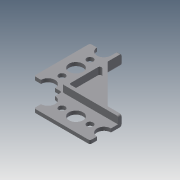
# Autodesk Inventor part: Деталь
Saved by Autodesk Inventor 2014 (Build 180170000, 170)
## iProperties
Created: 2015-11-19
Part Number: Деталь
Material: Типовые
Document SubType Name: Modeling
Designer: 151-362
Density: 1 g/cm^3
Appearance: По умолчанию
Author: 151-362
Autodesk Inventor part; units mm, degrees
ref_plane "YZ Plane" through (0, 0, 0) normal (1, 0, 0) x (0, 1, 0)
ref_plane "XZ Plane" through (0, 0, 0) normal (0, 1, 0) x (-1, 0, 0)
sketch "Эскиз1" plane through (0, 0, 0) normal (0, 0, 1) x (1, 0, 0)
  line L0 (0, 16) -> (0, 48)
  line L1 (0, 48) -> (4, 48)
  arc A0 (4, 48) -> (12, 48) centre (8, 48) ccw
  line L2 (12, 48) -> (18, 48)
  line L3 (18, 48) -> (18, 40)
  line L4 (18, 40) -> (40, 18)
  line L5 (40, 18) -> (48, 18)
  line L6 (48, 18) -> (48, 12)
  arc A1 (48, 12) -> (48, 4) centre (48, 8) ccw
  line L7 (48, 4) -> (48, 0)
  line L8 (48, 0) -> (16, 0)
  line L9 (16, 0) -> (16, 4)
  arc A2 (16, 4) -> (16, 12) centre (16, 8) ccw
  line L10 (16, 12) -> (16, 16)
  line L11 (16, 16) -> (12, 16)
  arc A3 (12, 16) -> (4, 16) centre (8, 16) ccw
  line L12 (0, 16) -> (4, 16)
  circle A4 centre (8, 24) radius 1.85
  circle A5 centre (8, 32) radius 4
  circle A6 centre (8, 40) radius 1.85
  circle A7 centre (40, 8) radius 1.85
  circle A8 centre (32, 8) radius 4
  circle A9 centre (24, 8) radius 1.85
  constraints: 26 end point, 10 centre point, 8 point on circle
extrude "Выдавливание1" add sketch "Эскиз1" along normal blind 2
fillet "Сопряжение1" radius 1 8 edges at (0, 48, 1) (18, 44, 0) (29, 29, 0) (44, 18, 0) (48, 0, 1) (16, 0, 1) (16, 16, 1) (0, 16, 1)
ref_plane "РабПлоскость1" through (0, 0, 2) normal (0, 0, 1) x (1, 0, 0)
sketch "Эскиз2" plane through (0, 0, 2) normal (0, 0, 1) x (1, 0, 0)
  line L0 (16, 16) -> (16, 48)
  line L1 (16, 48) -> (18, 48)
  line L2 (18, 48) -> (18, 40)
  line L3 (18, 40) -> (40, 18)
  line L4 (40, 18) -> (48, 18)
  line L5 (48, 18) -> (48, 16)
  line L6 (16, 16) -> (48, 16)
  line L7 (18, 18) -> (18, 37)
  line L8 (18, 37) -> (37, 18)
  line L9 (18, 18) -> (37, 18)
  constraints: 20 end point
extrude "Выдавливание2" add sketch "Эскиз2" along normal blind 4
fillet "Сопряжение2" radius 1 8 edges at (37, 18, 4) (18, 37, 4) (18, 18, 4) (16, 16, 4) (48, 17, 6) (17, 48, 6) (17.7071, 39.8787, 0.2929) (39.8787, 17.7071, 0.2929)
